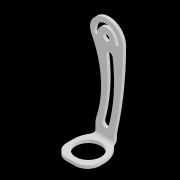
# Autodesk Inventor part: PullSolenoidArmBracket
Saved by Autodesk Inventor 2020 (Build 240168000, 168)
## iProperties
Created: 2020-04-24
Part Number: PullSolenoidArmBracket
Material: Generic
Document SubType Name: Sheet Metal
Designer: valer
Density: 1 g/cm^3
Sheet Metal Rule: Default
Appearance: Default
Flat Pattern Width: 3.38667 cm
Flat Pattern Length: 14.253 cm
Flat Pattern Area: 48.2703 cm^2
Sheet Metal Width: 1.333 in
Sheet Metal Length: 5.611 in
Sheet Metal Area: 7.482 in^2
Author: valer
Autodesk Inventor part; units mm, degrees
ref_plane "YZ Plane" through (0, 0, 0) normal (1, 0, 0) x (0, 1, 0)
ref_plane "XZ Plane" through (0, 0, 0) normal (0, 1, 0) x (-1, 0, 0)
ref_plane "XY Plane" through (0, 0, 0) normal (0, 0, 1) x (1, 0, 0)
sketch "ForearmMount" plane through (0, 0, 0) normal (0, 0, 1) x (1, 0, 0)
  circle A0 centre (0, 0) radius 3.175
  circle A1 centre (0, 0) radius 16.9333
  line L0 (-16.9333, 0) -> (-16.9333, -88.9)
  line L1 (-16.9333, -88.9) -> (16.9333, -88.9)
  line L2 (16.9333, -88.9) -> (16.9333, 0)
  dimension "d0" = 6.35
  dimension "d1" = 33.8667
  dimension "d2" = 88.9
  measures "d0" diameter of A0
  measures "d1" diameter of A1
  measures "d2" distance of L0.start L0.end
extrude "Plate1" add sketch "ForearmMount" along normal blind 3.048
sketch "Sketch2" plane through (16.9333, -88.9, 3.048) normal (0, -1, 0) x (1, 0, 0)
  line L0 (-33.8667, 0) -> (0, 0)
  line L1 (0, 0) -> (0, 35.8987)
  line L2 (0, 35.8987) -> (-33.8667, 35.8987)
  line L3 (-33.8667, 35.8987) -> (-33.8667, 0)
  constraints: 6 end point, 1 horizontal, 1 perpendicular, 1 vertical
edge flange "SolenoidMountFeature" height 38.9467 angle 90 thickness 3.048 bend radius 3.048 thickness toward (0, -1, 0) relief straight relief width 3.048 relief depth 1.524 edges at (0, -88.9, 3.048) wall of the first edge with corners at (-16.9333, -88.9, 3.048) (16.9333, -88.9, 3.048) (16.9333, -88.9, 38.9467) (-16.9333, -88.9, 38.9467)
bend "Bend1"
corner "Corner1"
sketch "SolenoidMountHole" plane through (-16.9333, -88.9, 38.9467) normal (0, 1, 0) x (1, 0, 0)
  line L0 (0, 0) -> (33.8667, 0) projected
  circle A0 centre (16.9333, 17.78) radius 12.7
  line L1 (16.9333, 17.78) -> (16.9333, 0) construction
  line L2 (0, 0) -> (33.8667, 0) projected
  point P0 (16.9333, 38.9467)
  dimension "d14" = 25.4
  dimension "d15" = 17.78
  constraints: 2 end point, 1 centre point, 1 midpoint
  measures "d14" diameter of A0
  measures "d15" distance of L1.start L1.end
extrude "SolenoidMountHoleFeature" cut sketch "SolenoidMountHole" against normal blind 25.4
sketch "GenerativeDesign" plane through (0, 0, 3.048) normal (0, 0, 1) x (1, 0, 0)
  line L0 (16.9333, 0) -> (16.9333, -85.852) projected
  arc A0 (16.9333, 0) -> (-16.9333, 0) centre (0, 0) ccw construction
  arc A1 (-10.9218, -76.4973) -> (-16.9333, 0) centre (-96.2208, -44.7156) ccw
  arc A2 (7.6155, -81.798) -> (16.9333, 0) centre (-346.7625, 0) ccw
  arc A3 (-0.8927, -75.6398) -> (3.2008, -14.3442) centre (-150.7871, -34.8448) ccw construction
  arc A4 (2.2931, -76.5069) -> (6.4737, -13.9085) centre (-150.7871, -34.8448) ccw
  arc A5 (-4.0786, -74.7728) -> (-0.072, -14.7799) centre (-150.7871, -34.8448) ccw
  arc A6 (-4.0786, -74.7728) -> (2.2931, -76.5069) centre (-0.8927, -75.6398) ccw
  arc A7 (6.4737, -13.9085) -> (-0.072, -14.7799) centre (3.2008, -14.3442) ccw
  line L1 (-10.9218, -76.4973) -> (-10.9218, -88.9)
  line L2 (-16.9333, -88.9) -> (16.9333, -88.9) projected
  line L3 (7.6155, -81.798) -> (7.6155, -88.9)
  line L4 (-16.9333, -85.852) -> (-16.9333, 0) projected
  line L5 (-16.9333, -85.852) -> (16.9333, -85.852) projected
  line L6 (0, 6.35) -> (0, 0) construction
  line L7 (-16.9333, -85.852) -> (16.9333, -85.852) projected
  line L8 (16.9333, 0) -> (16.9333, -85.852) projected
  arc A8 (16.9333, 0) -> (-16.9333, 0) centre (0, 0) ccw construction
  line L9 (-16.9333, -85.852) -> (-16.9333, 0) projected
  circle A9 centre (0, 0) radius 3.175 construction
  arc A10 (10.4888, -0.2887) -> (-10.4888, -0.2887) centre (0, 0) ccw construction
  arc A11 (12.101, -0.3331) -> (-12.101, -0.3331) centre (0, 0) ccw
  arc A12 (8.8767, -0.2443) -> (-8.8767, -0.2443) centre (0, 0) ccw
  arc A13 (8.8767, -0.2443) -> (12.101, -0.3331) centre (10.4888, -0.2887) ccw
  arc A14 (-12.101, -0.3331) -> (-8.8767, -0.2443) centre (-10.4888, -0.2887) ccw
  point P0 (7.6155, -85.852)
  point P1 (-10.9218, -85.852)
  dimension "d28" = 6.35
  constraints: 24 point on circle, 12 centre point, 9 tangent, 6 end point, 2 point on line, 2 vertical, 1 concentric, 1 perpendicular
  measures "d28" distance of point (0, 0) L6.start
extrude "GenerativeDesignFeature" cut sketch "GenerativeDesign" against normal blind 25.4 contours L5 L4 A1 L1 | L0 L5 L3 A2 | A6 A5 A7 A4 | A13 A12 A14 A11
fillet "Fillets1Feature" radius 12.7 3 edges at (-16.9333, -90.424, 38.9467) (16.9333, -90.424, 38.9467) (-16.9333, 0, 1.524)
sketch "MountShape" plane through (-16.9333, -85.852, 0) normal (0, 1, 0) x (1, 0, 0)
  line L0 (0, -3.048) -> (6.0115, -3.048) projected
  line L1 (24.5488, -3.048) -> (33.8667, -3.048) projected
  line L2 (0, -6.096) -> (0, -26.2467) projected
  line L3 (33.8667, -6.096) -> (33.8667, -26.2467) projected
  line L4 (6.0115, -3.048) -> (6.0115, 0) projected
  line L5 (6.0115, -3.048) -> (0, -10.0806)
  line L6 (24.5488, -3.048) -> (33.8667, -10.0806)
  line L7 (33.8667, -3.048) -> (33.8667, -6.096) projected
  line L8 (33.8667, -10.0806) -> (33.8667, -3.048)
  line L9 (0, -3.048) -> (0, -6.096) projected
  line L10 (0, -3.048) -> (0, -10.0806)
  line L11 (0, 0) -> (0, -3.048) projected
  line L12 (6.0115, 0) -> (0, 0) projected
  line L13 (24.5488, -3.048) -> (24.5488, 0) projected
  line L14 (33.8667, 0) -> (24.5488, 0) projected
  line L15 (33.8667, -3.048) -> (33.8667, 0) projected
  point P0 (16.9333, 0)
  constraints: 8 end point, 2 point on line, 1 collinear, 1 vertical
extrude "MountShapeFeature" cut sketch "MountShape" against normal mid plane 25.4
delete faces "Delete1" heal yes whole lump no faces at (8.8723, -73.152, 2.032)
fillet "Fillets2Feature" radius 25.4 2 edges at (-16.9333, -90.424, 10.0806) (16.9333, -90.424, 10.0806)
fillet "Fillets3Feature" radius 25.4 2 edges at (7.6155, -81.798, 1.524) (-10.9218, -76.4973, 1.524)
equation "\"d3\" = Thickness"
equation "\"d4\" = BendReliefWidth"
equation "\"d5\" = BendReliefDepth"
equation "\"d6\" = MinimumRemnant"
equation "\"d7\" = TransitionRadius"
equation "\"d10\" = BendRadius"
equation "\"d11\" = CornerReliefSize"
equation "\"d12\" = GapSize"
equation "\"d13\" = JacobiRadiusSize"
equation "\"BendRadius\" = Thickness"
equation "\"BendReliefWidth\" = Thickness"
equation "\"BendReliefDepth\" = 0.5 * Thickness"
equation "\"CornerReliefSize\" = 4 * Thickness"
equation "\"MinimumRemnant\" = 2 * Thickness"
equation "\"TransitionRadius\" = BendRadius"
equation "\"JacobiRadiusSize\" = BendRadius"
equation "\"GapSize\" = Thickness"
equation "\"Thickness\" = 3.048"
body "Solid1"
